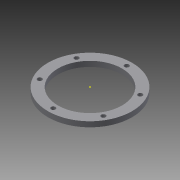
# Autodesk Inventor part: middle plate
Saved by Autodesk Inventor 2015 (Build 190159000, 159)
## iProperties
Created: 2015-02-28
Part Number: middle plate
Material: Generic
Document SubType Name: Modeling
Designer: Qiuyang
Density: 1 g/cm^3
Appearance: Default
Author: Qiuyang
Autodesk Inventor part; units mm, degrees
ref_plane "YZ Plane" through (0, 0, 0) normal (1, 0, 0) x (0, 1, 0)
ref_plane "XZ Plane" through (0, 0, 0) normal (0, 1, 0) x (-1, 0, 0)
ref_plane "XY Plane" through (0, 0, 0) normal (0, 0, 1) x (1, 0, 0)
sketch "Sketch4" plane through (0, 0, 0) normal (0, 1, 0) x (-1, 0, 0)
  circle A0 centre (0, 0) radius 38.735
  circle A1 centre (0, 0) radius 50.8
  dimension "d9" = 77.47
  dimension "d10" = 101.6
  constraints: 2 centre point, 2 coincident
  measures "d9" diameter of A0
  measures "d10" diameter of A1
extrude "Extrusion2" add sketch "Sketch4" along normal blind 6.35
sketch "Sketch5" plane through (0, 6.35, 0) normal (0, 1, 0) x (1, 0, 0)
  circle A0 centre (0, -44.45) radius 2.667
  circle A1 centre (38.4948, -22.225) radius 2.667
  circle A2 centre (38.4948, 22.225) radius 2.667
  circle A3 centre (0, 44.45) radius 2.667
  circle A4 centre (-38.4948, 22.225) radius 2.667
  circle A5 centre (-38.4948, -22.225) radius 2.667
  point P0 (0, 0)
  dimension "d13" = 5.334
  dimension "d16" = 360
  constraints: 6 centre point, 13 other
  measures "d13" diameter of A0
extrude "Extrusion3" cut sketch "Sketch5" against normal blind 6.35
sketch "Sketch6" plane through (0, 6.35, 0) normal (0, 1, 0) x (1, 0, 0)
  point P0 (0, 0)
body "Solid2"
